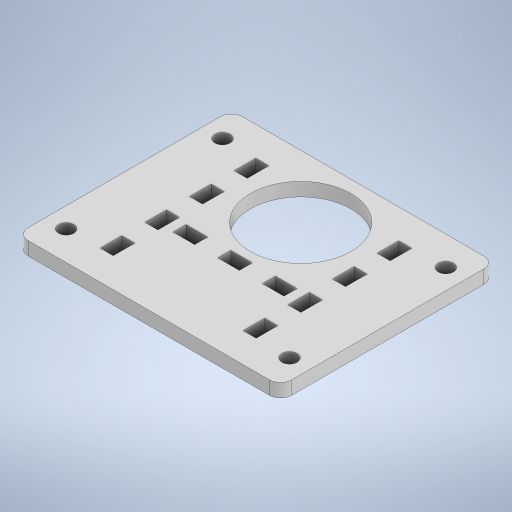
# Autodesk Inventor part: Module_base_MFC
Saved by Autodesk Inventor 2023 (Build 270158000, 158)
## iProperties
Created: 2022-10-28
Part Number: Module_base_MFC
Material: Generic
Document SubType Name: Modeling
Designer: incep
Density: 1 g/cm^3
Appearance: Default
Author: incep
Autodesk Inventor part; units mm, degrees
ref_plane "YZ Plane" through (0, 0, 0) normal (1, 0, 0) x (0, 1, 0)
ref_plane "XZ Plane" through (0, 0, 0) normal (0, 1, 0) x (-1, 0, 0)
ref_plane "XY Plane" through (0, 0, 0) normal (0, 0, 1) x (1, 0, 0)
sketch "Sketch1" plane through (0, 0, 0) normal (0, 1, 0) x (-1, 0, 0)
  line L0 (54, -48) -> (-54, -48)
  line L1 (-59, -43) -> (-59, 43)
  line L2 (-54, 48) -> (54, 48)
  line L3 (59, 43) -> (59, -43)
  line L4 (50, -35) -> (-50, -35) construction
  line L5 (-50, -35) -> (-50, 35) construction
  line L6 (-50, 35) -> (50, 35) construction
  line L7 (50, 35) -> (50, -35) construction
  arc A0 (59, 43) -> (54, 48) centre (54, 43) ccw
  arc A1 (-54, 48) -> (-59, 43) centre (-54, 43) ccw
  arc A2 (-59, -43) -> (-54, -48) centre (-54, -43) ccw
  arc A3 (54, -48) -> (59, -43) centre (54, -43) ccw
  circle A4 centre (50, -35) radius 3.4
  circle A5 centre (50, 35) radius 3.4
  circle A6 centre (-50, -35) radius 3.4
  circle A7 centre (-50, 35) radius 3.4
  line L8 (0, -20) -> (0, 20) construction
  line L9 (25, -20) -> (25, 20) construction
  line L10 (-25, 20) -> (-25, -20) construction
  arc A8 (-25, -20) -> (25, -20) centre (0, -20) ccw construction
  arc A9 (25, 20) -> (-25, 20) centre (0, 20) ccw construction
  circle A10 centre (0, -20) radius 22.5
  circle A11 centre (50, -35) radius 9.5 construction
  circle A12 centre (-50, -35) radius 9.5 construction
  circle A13 centre (50, 35) radius 9.5 construction
  circle A14 centre (-50, 35) radius 9.5 construction
  line L11 (35, -35) -> (29, -35) construction
  line L12 (29, -35) -> (29, 35) construction
  line L13 (29, 35) -> (35, 35) construction
  line L14 (35, 35) -> (35, -35) construction
  line L15 (35, 6.4) -> (-35, 6.4) construction
  line L16 (-35, 12.4) -> (35, 12.4) construction
  line L17 (35, 12.4) -> (35, 6.4) construction
  line L18 (-25, -20) -> (-25, 20) construction
  line L19 (4.85, 6.475) -> (-4.85, 6.475)
  line L20 (-4.85, 6.475) -> (-4.85, 12.325)
  line L21 (-4.85, 12.325) -> (4.85, 12.325)
  line L22 (4.85, 12.325) -> (4.85, 6.475)
  line L23 (0, 6.4) -> (0, 12.4) construction
  line L24 (34.925, -34.85) -> (29.075, -34.85)
  line L25 (29.075, -34.85) -> (29.075, -25.15)
  line L26 (29.075, -25.15) -> (34.925, -25.15)
  line L27 (34.925, -25.15) -> (34.925, -34.85)
  line L28 (34.925, -14.85) -> (29.075, -14.85)
  line L29 (34.925, -5.15) -> (34.925, -14.85)
  line L30 (29.075, -5.15) -> (34.925, -5.15)
  line L31 (29.075, -14.85) -> (29.075, -5.15)
  line L32 (34.925, 5.15) -> (29.075, 5.15)
  line L33 (34.925, 14.85) -> (34.925, 5.15)
  line L34 (29.075, 14.85) -> (34.925, 14.85)
  line L35 (29.075, 5.15) -> (29.075, 14.85)
  line L36 (34.925, 25.15) -> (29.075, 25.15)
  line L37 (34.925, 34.85) -> (34.925, 25.15)
  line L38 (29.075, 34.85) -> (34.925, 34.85)
  line L39 (29.075, 25.15) -> (29.075, 34.85)
  line L40 (-35, -35) -> (-29, -35) construction
  line L41 (-29, -35) -> (-29, 35) construction
  line L42 (-29, 35) -> (-35, 35) construction
  line L43 (-35, 35) -> (-35, -35) construction
  line L44 (-35, 12.4) -> (-35, 6.4) construction
  line L45 (-34.925, -34.85) -> (-29.075, -34.85)
  line L46 (-29.075, -34.85) -> (-29.075, -25.15)
  line L47 (-29.075, -25.15) -> (-34.925, -25.15)
  line L48 (-34.925, -25.15) -> (-34.925, -34.85)
  line L49 (-34.925, -14.85) -> (-29.075, -14.85)
  line L50 (-34.925, -5.15) -> (-34.925, -14.85)
  line L51 (-29.075, -5.15) -> (-34.925, -5.15)
  line L52 (-29.075, -14.85) -> (-29.075, -5.15)
  line L53 (-34.925, 5.15) -> (-29.075, 5.15)
  line L54 (-34.925, 14.85) -> (-34.925, 5.15)
  line L55 (-29.075, 14.85) -> (-34.925, 14.85)
  line L56 (-29.075, 5.15) -> (-29.075, 14.85)
  line L57 (-34.925, 25.15) -> (-29.075, 25.15)
  line L58 (-34.925, 34.85) -> (-34.925, 25.15)
  line L59 (-29.075, 34.85) -> (-34.925, 34.85)
  line L60 (-29.075, 25.15) -> (-29.075, 34.85)
  line L61 (24.85, 6.475) -> (15.15, 6.475)
  line L62 (24.85, 12.325) -> (24.85, 6.475)
  line L63 (20, 6.4) -> (20, 12.4) construction
  line L64 (15.15, 12.325) -> (24.85, 12.325)
  line L65 (15.15, 6.475) -> (15.15, 12.325)
  line L66 (-15.15, 6.475) -> (-24.85, 6.475)
  line L67 (-15.15, 12.325) -> (-15.15, 6.475)
  line L68 (-20, 6.4) -> (-20, 12.4) construction
  line L69 (-24.85, 12.325) -> (-15.15, 12.325)
  line L70 (-24.85, 6.475) -> (-24.85, 12.325)
  line L71 (4.85, 6.475) -> (-4.85, 6.475)
  line L72 (4.85, 12.325) -> (4.85, 6.475)
  line L73 (0, 6.4) -> (0, 12.4) construction
  line L74 (-4.85, 12.325) -> (4.85, 12.325)
  line L75 (-4.85, 6.475) -> (-4.85, 12.325)
  point P0 (0, 0)
  point P1 (-59, 0)
  point P2 (0, -48)
  point P3 (0, -35)
  point P4 (-50, 0)
  point P5 (0, 0)
  point P6 (32, -35)
  point P7 (-4.85, 9.4)
  point P8 (4.85, 9.4)
  point P9 (0, 6.475)
  point P10 (32, -25.15)
  point P11 (32, -30)
  point P12 (29.075, -30)
  point P13 (32, -34.85)
  point P14 (32, -35)
  point P15 (29, 0)
  point P16 (32, -14.85)
  point P17 (32, -5.15)
  point P18 (29.075, -10)
  point P19 (32, -10)
  point P20 (32, 5.15)
  point P21 (32, 14.85)
  point P22 (29.075, 10)
  point P23 (32, 10)
  point P24 (32, 25.15)
  point P25 (32, 34.85)
  point P26 (29.075, 30)
  point P27 (32, 30)
  point P28 (-32, -35)
  point P29 (-32, -25.15)
  point P30 (-32, -30)
  point P31 (-29.075, -30)
  point P32 (-32, -34.85)
  point P33 (-32, -35)
  point P34 (-29, 0)
  point P35 (-32, -14.85)
  point P36 (-32, -5.15)
  point P37 (-29.075, -10)
  point P38 (-32, -10)
  point P39 (-32, 5.15)
  point P40 (-32, 14.85)
  point P41 (-29.075, 10)
  point P42 (-32, 10)
  point P43 (-32, 25.15)
  point P44 (-32, 34.85)
  point P45 (-29.075, 30)
  point P46 (-32, 30)
  point P47 (35, 9.4)
  point P48 (35, 0)
  point P49 (20, 6.475)
  point P50 (24.85, 9.4)
  point P51 (15.15, 9.4)
  point P52 (-20, 6.475)
  point P53 (-15.15, 9.4)
  point P54 (-24.85, 9.4)
  point P55 (0, 6.475)
  point P56 (4.85, 9.4)
  point P57 (-4.85, 9.4)
  dimension "d0" = 96
  dimension "d1" = 118
  dimension "d2" = 70
  dimension "d3" = 100
  dimension "d4" = 5
  dimension "d5" = 6.8
  dimension "d6" = 6.8
  dimension "d8" = 6.8
  dimension "d10" = 6.8
  dimension "d13" = 25
  dimension "d14" = 40
  dimension "d17" = 45
  dimension "d19" = 19
  dimension "d22" = 100
  dimension "d25" = 70
  dimension "d28" = 6
  dimension "d29" = 6
  dimension "d30" = 26.4
  dimension "d31" = 15
  dimension "d41" = 5.85
  dimension "d42" = 9.7
  dimension "d54" = 5.85
  dimension "d55" = 9.7
  dimension "d56" = 30
  dimension "d59" = 20
  dimension "d64" = 9.4
  dimension "d67" = 20
  dimension "d70" = 20
  constraints: 154 end point, 39 symmetric about line, 17 midpoint, 15 centre point, 12 parallel, 12 point on circle, 12 tangent, 9 horizontal, 6 coincident, 6 horizontal alignment, 6 vertical alignment, 5 perpendicular, 3 equal radius, 3 vertical, 1 collinear, 84 other
  measures "d0" distance between parallel lines of L2 L0
  measures "d1" distance between parallel lines of L1 L3
  measures "d2" distance between parallel lines of L6 L4
  measures "d3" distance between parallel lines of L7 L5
  measures "d4" radius of A0
  measures "d5" diameter of A4
  measures "d6" diameter of A5
  measures "d8" diameter of A6
  measures "d10" diameter of A7
  measures "d13" radius of A8
  measures "d14" distance of L8.end L8.start
  measures "d17" diameter of A10
  measures "d19" diameter of A11
  measures "d22" distance of A11.centre A12.centre
  measures "d25" distance of A11.centre A13.centre
  measures "d28" distance between parallel lines of L12 L14
  measures "d29" distance between parallel lines of L16 L15
  measures "d30" distance of L23.start L8.start
  measures "d31" distance of L11.start L4.start
  measures "d41" distance between parallel lines of L21 L19
  measures "d42" distance from line of L20 point (4.85, 9.4)
  measures "d54" distance between parallel lines of L25 L27
  measures "d55" distance from line of point (32, -25.15) L24
  measures "d56" vertical distance of point (29, 0) point (32, -30)
  measures "d59" distance of L24.start L28.start
  measures "d64" distance of point (35, 9.4) point (35, 0)
  measures "d67" distance of L23.start L63.start
  measures "d70" distance of L23.start L68.start
extrude "Extrusion1" add sketch "Sketch1" along normal blind 6
equation "\"d0\" = moduleHeight"
equation "\"d1\" = moduleWidth"
equation "\"d2\" = moduleMountH"
equation "\"d3\" = moduleMountW"
equation "\"d4\" = moduleCornerR"
equation "\"d5\" = moduleMountD"
equation "\"d6\" = moduleMountD"
equation "\"d8\" = moduleMountD"
equation "\"d10\" = moduleMountD"
equation "\"d13\" = moduleOpeningR"
equation "\"d14\" = moduleOpeningH"
equation "\"d17\" = openingMFC"
equation "\"d19\" = moduleMountClearance"
equation "\"d28\" = thickness"
equation "\"d29\" = thickness"
equation "\"d30\" = 0.5 * actuatorH + thickness"
equation "\"d31\" = supportSpacingFromMounting"
equation "\"d41\" = fingerholeH"
equation "\"d42\" = fingerholeW"
equation "\"d54\" = fingerholeH"
equation "\"d55\" = fingerholeW"
equation "\"d56\" = 1.5 * fingerSpacing"
equation "\"d15\" = thickness"
equation "\"moduleWidth\" = 118"
equation "\"moduleHeight\" = 96"
equation "\"moduleMountW\" = 100"
equation "\"moduleMountH\" = 70"
equation "\"moduleMountD\" = 6.8"
equation "\"moduleCornerR\" = 5"
equation "\"moduleOpeningR\" = 25"
equation "\"moduleOpeningH\" = 40"
equation "\"thickness\" = 6"
equation "\"kerf\" = 0.15"
equation "\"fingerholeW\" = fingerW - 2 * kerf"
equation "\"fingerholeH\" = thickness - kerf"
equation "\"moduleMountClearance\" = 19"
equation "\"actuatorW\" = 28"
equation "\"actuatorH\" = 40.8"
equation "\"openingMFC\" = 45"
equation "\"supportXW\" = -2 * thickness + moduleMountW - 2 * supportSpacingFromMounting + kerf"
equation "\"supportSpacingFromMounting\" = 15"
equation "\"supportsCTCZ\" = 9.4"
equation "\"fingerW\" = 10"
equation "\"fingerSpacing\" = 20"
body "Solid1"
